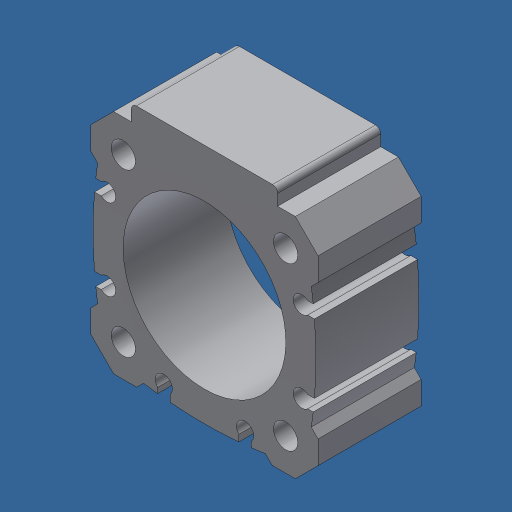
# Autodesk Inventor part: EXTRUSION, CYLINDER, ALUMINIUM, PHD, 40MM
Saved by Autodesk Inventor 2024.3 (Build 283343000, 343)
## iProperties
Manager: _
Category: _
ILogicPurgeVersion: 2.2.20.20
OnSaveVersion: 2.2.20.20
Shininess: 64.0
Angle Display Precision: 2
Document Length Units: 11272
Document Angle Units: 11279
Document Time Units: 11290
Document Mass Units: 11286
Document Length Units Precision: 3
Document Angle Units Precision: 2
Part Number: EXTRUSION, CYLINDER, ALUMINIUM, PHD, 40MM
Material: Extrusion, Aluminum, PHD, 40MM
Document SubType Name: Modeling
Created: 2023-11-08
Designer: -
Manufacturer: Standard
Standards Organization: Custom
Checked By: 00
Engr Approved By: _
User Status: Work In Process
Description: EXTRUSION, CYLINDER, ALUMINIUM, PHD, 40MM
Density: 2.71 g/cm^3
Mass: 113.203 g
Surface Area: 155.436 cm^2
Volume: 41.7724 cm^3
Mfg Approved By: Stephen.Oerton
Appearance: Aluminum - Flat
Density: 0.0
Volumn: 0.0
Area: 0.0
PropertySet Name: Model Information
Control State: 0
Master: False
Checked Out: False
CN_MASS: 0.11
CN_SERVICEABLE: _
CL_runCount: 0
FIRST_DESCRIPTION: _
SECOND_DESCRIPTION: _
THIRD_DESCRIPTION: _
ModelCat: Uncategorized
Revision Number: A
Subject: _
Author: -
Keywords: -
Autodesk Inventor part; units mm, degrees
ref_plane "YZ Plane" through (0, 0, 0) normal (1, 0, 0) x (0, 1, 0)
ref_plane "XZ Plane" through (0, 0, 0) normal (0, 1, 0) x (-1, 0, 0)
ref_plane "XY Plane" through (0, 0, 0) normal (0, 0, 1) x (1, 0, 0)
sketch "Sketch1" plane through (0, 0, 0) normal (0, 0, 1) x (1, 0, 0)
  line L0 (0, 98.7215) -> (0, -37.7435) projected
  line L1 (-83.3748, 0) -> (111.1664, 0) projected
  line L2 (-16.764, 32.004) -> (0, 32.004)
  line L3 (0, 0) -> (0, 34.9655) construction
  line L4 (-18.034, 30.734) -> (-18.034, 27.991)
  arc A0 (-16.764, 32.004) -> (-18.034, 30.734) centre (-16.764, 30.734) ccw
  line L5 (-18.034, 27.991) -> (-22.397, 27.991)
  line L6 (-22.397, 27.991) -> (-28, 22.388)
  line L7 (-28, 22.388) -> (-28, 16.697)
  line L8 (-28, 16.697) -> (-26.314, 15.011)
  arc A1 (-25.4656, 8.472) -> (-25.4646, 11.545) centre (-24.003, 10.008) ccw
  line L9 (-26.7932, 11.545) -> (-25.4646, 11.545)
  line L10 (-27.1122, 8.472) -> (-25.4656, 8.472)
  arc A2 (-26.314, 15.011) -> (-26.7932, 11.545) centre (69.479, 0) ccw
  arc A3 (-25.4646, -11.545) -> (-25.4656, -8.472) centre (-24.003, -10.008) ccw
  line L11 (-27.1122, -8.472) -> (-25.4656, -8.472)
  line L12 (-26.7932, -11.545) -> (-25.4646, -11.545)
  arc A4 (-27.1122, 8.472) -> (-27.1122, -8.472) centre (69.479, 0) ccw
  line L13 (-26.314, -15.011) -> (-28, -16.697)
  line L14 (-28, -16.697) -> (-28, -22.393)
  line L15 (-28, -22.393) -> (-22.397, -27.996)
  line L16 (-22.397, -27.996) -> (-16.693, -27.996)
  line L17 (-16.693, -27.996) -> (-15.011, -26.314)
  arc A5 (-26.7932, -11.545) -> (-26.314, -15.011) centre (69.479, 0) ccw
  arc A6 (-8.472, -25.4656) -> (-11.545, -25.4646) centre (-10.008, -24.003) ccw
  line L18 (-11.545, -25.4646) -> (-11.545, -26.7932)
  line L19 (-8.472, -25.4656) -> (-8.472, -27.1122)
  arc A7 (-15.011, -26.314) -> (-11.545, -26.7932) centre (0, 69.479) ccw
  arc A8 (-8.472, -27.1122) -> (0, -27.483) centre (0, 69.479) ccw
  arc A9 (0, 20.066) -> (0, -20.066) centre (0, 0) ccw
  line L20 (0, 32.004) -> (0, -27.483) construction
  circle A10 centre (-20, 20.003) radius 3
  circle A11 centre (-20, -20.003) radius 3
  line L21 (16.764, 32.004) -> (0, 32.004)
  line L22 (18.034, 30.734) -> (18.034, 27.991)
  arc A12 (18.034, 30.734) -> (16.764, 32.004) centre (16.764, 30.734) ccw
  line L23 (18.034, 27.991) -> (22.397, 27.991)
  line L24 (22.397, 27.991) -> (28, 22.388)
  line L25 (28, 22.388) -> (28, 16.697)
  line L26 (28, 16.697) -> (26.314, 15.011)
  arc A13 (25.4646, 11.545) -> (25.4656, 8.472) centre (24.003, 10.008) ccw
  line L27 (26.7932, 11.545) -> (25.4646, 11.545)
  line L28 (27.1122, 8.472) -> (25.4656, 8.472)
  arc A14 (26.7932, 11.545) -> (26.314, 15.011) centre (-69.479, 0) ccw
  arc A15 (25.4656, -8.472) -> (25.4646, -11.545) centre (24.003, -10.008) ccw
  line L29 (27.1122, -8.472) -> (25.4656, -8.472)
  line L30 (26.7932, -11.545) -> (25.4646, -11.545)
  arc A16 (27.1122, -8.472) -> (27.1122, 8.472) centre (-69.479, 0) ccw
  line L31 (26.314, -15.011) -> (28, -16.697)
  line L32 (28, -16.697) -> (28, -22.393)
  line L33 (28, -22.393) -> (22.397, -27.996)
  line L34 (22.397, -27.996) -> (16.693, -27.996)
  line L35 (16.693, -27.996) -> (15.011, -26.314)
  arc A17 (26.314, -15.011) -> (26.7932, -11.545) centre (-69.479, 0) ccw
  arc A18 (11.545, -25.4646) -> (8.472, -25.4656) centre (10.008, -24.003) ccw
  line L36 (11.545, -25.4646) -> (11.545, -26.7932)
  line L37 (8.472, -25.4656) -> (8.472, -27.1122)
  arc A19 (11.545, -26.7932) -> (15.011, -26.314) centre (0, 69.479) ccw
  arc A20 (0, -27.483) -> (8.472, -27.1122) centre (0, 69.479) ccw
  arc A21 (0, -20.066) -> (0, 20.066) centre (0, 0) ccw
  circle A22 centre (20, 20.003) radius 3
  circle A23 centre (20, -20.003) radius 3
  dimension "d0" = 69.479
  dimension "d2" = 69.479
  dimension "d4" = 32.004
  dimension "d5" = 18.034
  dimension "d6" = 2.54
  dimension "d7" = 27.991
  dimension "d8" = 135
  dimension "d9" = 28
  dimension "d10" = 4.363
  dimension "d11" = 16.697
  dimension "d12" = 135
  dimension "d13" = 10.008
  dimension "d14" = 24.003
  dimension "d15" = 4.242
  dimension "d16" = 11.545
  dimension "d17" = 8.472
  dimension "d18" = 96.962
  dimension "d19" = 10.008
  dimension "d20" = 4.242
  dimension "d21" = 8.472
  dimension "d22" = 11.545
  dimension "d23" = 96.962
  dimension "d24" = 15.011
  dimension "d26" = 45
  dimension "d27" = 28
  dimension "d28" = 22.393
  dimension "d29" = 135
  dimension "d30" = 22.397
  dimension "d31" = 16.693
  dimension "d32" = 135
  dimension "d33" = 96.962
  dimension "d34" = 10.008
  dimension "d35" = 24.003
  dimension "d36" = 4.242
  dimension "d38" = 11.545
  dimension "d39" = 8.472
  dimension "d40" = 96.962
  dimension "d41" = 96.962
  dimension "d42" = 40.132
  dimension "d43" = 20
  dimension "d44" = 20.003
  dimension "d45" = 6
  dimension "d46" = 20.003
  dimension "d47" = 6
  constraints: 72 end point, 40 point on circle, 32 symmetric about line, 24 centre point, 7 parallel, 6 perpendicular, 6 point on line, 3 vertical alignment, 2 tangent, 1 coincident, 1 horizontal alignment, 29 other
  measures "d0" distance of A2.centre L3.start
  measures "d2" horizontal distance of A7.centre A2.centre
  measures "d4" distance from line of L3.start L2
  measures "d5" distance between parallel lines of L3 L4
  measures "d6" diameter of A0
  measures "d7" distance between parallel lines of L1 L5
  measures "d8" angle of L5 L6
  measures "d9" distance between parallel lines of L3 L7
  measures "d10" distance of L4.end L5.end
  measures "d11" distance from line of L1 L7.end
  measures "d12" angle of L8 L7
  measures "d13" distance from line of A1.centre L1
  measures "d14" distance from line of L3 A1.centre
  measures "d15" diameter of A1
  measures "d16" distance between parallel lines of L1 L9
  measures "d17" distance between parallel lines of L1 L10
  measures "d18" radius of A2
  measures "d19" distance from line of A3.centre L1
  measures "d20" diameter of A3
  measures "d21" distance between parallel lines of L11 L1
  measures "d22" distance between parallel lines of L12 L1
  measures "d23" radius of A4
  measures "d24" distance from line of L1 L13.start
  measures "d26" angle of L1 L13
  measures "d27" distance between parallel lines of L0 L14
  measures "d28" distance from line of L14.end L1
  measures "d29" angle of L15 L14
  measures "d30" distance from line of L0 L15.end
  measures "d31" distance from line of L0 L16.end
  measures "d32" angle of L17 L16
  measures "d33" radius of A5
  measures "d34" distance from line of L0 A6.centre
  measures "d35" distance from line of L1 A6.centre
  measures "d36" diameter of A6
  measures "d38" distance between parallel lines of L0 L18
  measures "d39" distance between parallel lines of L0 L19
  measures "d40" radius of A7
  measures "d41" radius of A8
  measures "d42" diameter of A9
  measures "d43" distance from line of L0 A11.centre
  measures "d44" distance from line of L1 A11.centre
  measures "d45" diameter of A11
  measures "d46" distance from line of L1 A10.centre
  measures "d47" diameter of A10
extrude "PHD, 40MM" add sketch "Sketch1" against normal blind 25.4 contours L21 A12 L22 L23 L24 L25 L26 A14 L27 A13 L28 A16 L1 A21 L0 | L0 A9 L1 A4 L10 A1 L9 A2 L8 L7 L6 L5 L4 A0 L2 | A9 L0 A8 L19 A6 L18 A7 L17 L16 L15 L14 L13 A5 L12 A3 L11 A4 L1 | L1 A16 L29 A15 L30 A17 L31 L32 L33 L34 L35 A19 L36 A18 L37 A20 L0 A21
equation "\"d19\" = d13"
equation "\"d20\" = d15"
equation "\"d21\" = d17"
equation "\"d22\" = d16"
equation "\"d46\" = d44"
equation "\"d47\" = d45"
